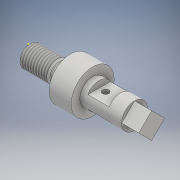
# Autodesk Inventor part: Семинр Курганова вал
Saved by Autodesk Inventor 2017 (Build 210142000, 142)
## iProperties
Part Number: Семинр Курганова вал
Material: Типовые
Document SubType Name: Modeling
Designer: Sasha
Density: 1 g/cm^3
Appearance: По умолчанию
Mass: 58.1575 g
Surface Area: 117.34 cm^2
Volume: 58.1575 cm^3
Author: Sasha
Autodesk Inventor part; units mm, degrees
ref_plane "YZ Plane" through (0, 0, 0) normal (1, 0, 0) x (0, 1, 0)
ref_plane "XZ Plane" through (0, 0, 0) normal (0, 1, 0) x (-1, 0, 0)
ref_plane "XY Plane" through (0, 0, 0) normal (0, 0, 1) x (1, 0, 0)
sketch "Эскиз1" plane through (0, 0, 0) normal (0, 0, 1) x (1, 0, 0)
  line L0 (0, 0) -> (0, 9.9999)
  line L1 (0, 9.9999) -> (27.2501, 9.9999)
  line L2 (27.2501, 9.9999) -> (29, 8.25)
  line L3 (29, 8.25) -> (35, 8.25)
  line L4 (35, 8.25) -> (35, 12.5)
  line L5 (35, 12.5) -> (39.3301, 20)
  line L6 (39.3301, 20) -> (60, 20)
  line L7 (60, 20) -> (60, 12)
  line L8 (60, 12) -> (99, 12)
  line L9 (99, 12) -> (99, 0)
  line L10 (99, 0) -> (0, 0)
  dimension "d1" = 45
  dimension "d2" = 30
  dimension "d3" = 6
  dimension "d4" = 35
  dimension "d7" = 24
  dimension "d8" = 19.9998
  dimension "d9" = 16.5
  dimension "d10" = 25
  dimension "d11" = 39
  dimension "d12" = 99
  dimension "d14" = 40
  constraints: 22 end point, 5 perpendicular, 2 parallel, 1 vertical
  measures "d1" angle of L1 L2
  measures "d2" angle of L5 L4
  measures "d3" distance of L2.end L3.end
  measures "d4" horizontal distance of L4.end L0.end
  measures "d7" diameter of L8 L10
  measures "d8" diameter of L1 L10
  measures "d9" diameter of L3 L10
  measures "d10" diameter of L4.end L10
  measures "d11" distance of L7.end L8.end
  measures "d12" distance of L9.end L0.start
  measures "d14" diameter of L6 L10
revolve "Вращение1" add sketch "Эскиз1" angle 360 about axis through (99, 0, 0) along (-1, 0, 0)
sketch "Эскиз2" plane through (99, 0, 0) normal (1, 0, 0) x (0, 0, -1)
  circle A0 centre (0, 0) radius 12 projected
  line L0 (12, 0) -> (0, 12)
  line L1 (0, 12) -> (-12.0353, -0.0353)
  line L2 (-12.0353, -0.0353) -> (-0.0353, -12.0353)
  line L3 (-0.0353, -12.0353) -> (12, 0)
  constraints: 8 end point, 2 parallel, 2 point on circle, 1 perpendicular
extrude "Выдавливание1" [suppressed]
sketch "Эскиз3" plane through (0, 0, 0) normal (0, 1, 0) x (-1, 0, 0)
  point P0 (0, 0)
sketch "Эскиз4" plane through (0, 0, 0) normal (0, 1, 0) x (-1, 0, 0)
  line L0 (-60, -12) -> (-99, -12) projected
  line L1 (-66, -12) -> (-86, -12)
  line L2 (-86, -12) -> (-86, -6.1869)
  line L3 (-86, -6.1869) -> (-66, -6.1869)
  line L4 (-66, -6.1869) -> (-66, -12)
  line L5 (-60, 12) -> (-99, 12) projected
  line L6 (-66, 12) -> (-86, 12)
  line L7 (-86, 12) -> (-86, 5.8131)
  line L8 (-86, 5.8131) -> (-66, 5.8131)
  line L9 (-66, 5.8131) -> (-66, 12)
  line L10 (-60, 20) -> (-60, -20) projected
  point P0 (0, 0)
  dimension "d18" = 6
  dimension "d19" = 6
  dimension "d20" = 20
  dimension "d21" = 12
  constraints: 16 end point, 5 parallel, 2 horizontal, 2 perpendicular, 2 point on line
  measures "d18" distance from line of L10 L1.start
  measures "d19" distance from line of L10 L6.start
  measures "d20" distance of L2.end L3.end
  measures "d21" distance of L7.end L2.end
extrude "Выдавливание2" cut sketch "Эскиз4" along normal through all both and the other way through all
sketch "Эскиз5" plane through (0, 0, 0) normal (0, 0, 1) x (1, 0, 0)
  line L0 (60, -12) -> (60, 12) projected
  line L1 (60, -20) -> (60, 20) projected
  line L2 (-21.8, 0) -> (130.8, 0) projected
  circle A0 centre (72, 0) radius 3
  point P0 (0, 0)
  dimension "d24" = 6
  dimension "d25" = 12
  constraints: 1 centre point, 1 point on line
  measures "d24" diameter of A0
  measures "d25" distance from line of L1 A0.centre
extrude "Выдавливание3" cut sketch "Эскиз5" along normal through all both and the other way through all
thread "Резьба1" size "M20x2.5" class "6g" standard "ISO Metric profile" full length
chamfer "Фаска1" distance 2.5 angle 45 1 edges at (0, -9.9999, 0)
fillet "Сопряжение1" radius 1 1 edges at (29, -8.25, 0)
fillet "Сопряжение2" radius 1.6 1 edges at (35, -8.25, 0)
sketch "Эскиз6" plane through (72, 0, 0) normal (0, 0, 1) x (1, 0, 0)
  point P0 (-72, 0)
sketch "Эскиз7" plane through (99, -8.4853, 8.4853) normal (0, 0, 1) x (1, 0, 0)
  point P0 (-99, 8.4853)
sketch "Эскиз8" plane through (99, 0, 0) normal (1, 0, 0) x (0, 0, -1)
  circle A0 centre (0, 0) radius 12 projected
  circle A1 centre (0, 0) radius 12 projected
  line L0 (12, -0.0264) -> (0, 12)
  line L1 (0, 12) -> (-12, 0.0264)
  line L2 (-12, 0.0264) -> (0, -12)
  line L3 (0, -12) -> (12, -0.0264)
  constraints: 8 end point, 3 point on circle, 2 parallel, 1 perpendicular, 2 other
extrude "Выдавливание4" add sketch "Эскиз8" along normal blind 16 contours L0 L3 L2 L1
